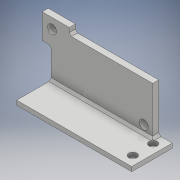
# Autodesk Inventor part: PingCover-y
Saved by Autodesk Inventor 2018 (Build 220112000, 112)
## iProperties
Created: 2018-08-25
Part Number: PingCover-y
Material: 一般
Document SubType Name: Modeling
Designer: shun2
Density: 1 g/cm^3
Appearance: 既定
Author: shun2
Autodesk Inventor part; units mm, degrees
ref_plane "YZ Plane" through (0, 0, 0) normal (1, 0, 0) x (0, 1, 0)
ref_plane "XZ Plane" through (0, 0, 0) normal (0, 1, 0) x (-1, 0, 0)
ref_plane "XY Plane" through (0, 0, 0) normal (0, 0, 1) x (1, 0, 0)
sketch "スケッチ1" plane through (0, 0, 0) normal (0, 0, 1) x (1, 0, 0)
  line L0 (0, 0) -> (51, 0)
  line L1 (51, 0) -> (51, 18)
  line L2 (51, 18) -> (0, 18)
  line L3 (0, 18) -> (0, 0)
  circle A0 centre (47, 13.5) radius 1.8
  circle A1 centre (47, 4.5) radius 1.8
  dimension "d0" = 51
  dimension "d1" = 18
  dimension "d4" = 3.6
  dimension "d5" = 13.5
  dimension "d6" = 4
  dimension "d7" = 3.6
  dimension "d8" = 4
  dimension "d9" = 4.5
  constraints: 8 end point, 2 centre point, 2 parallel, 1 horizontal, 1 perpendicular
  measures "d0" distance of L2.end L1.end
  measures "d1" distance of L1.end L0.end
  measures "d4" diameter of A0
  measures "d5" distance from line of L0 A0.centre
  measures "d6" distance from line of L1 A0.centre
  measures "d7" diameter of A1
  measures "d8" distance from line of L1 A1.centre
  measures "d9" distance from line of L0 A1.centre
extrude "押し出し2" add sketch "スケッチ1" along normal blind 2
sketch "スケッチ2" plane through (0, 0, 2) normal (0, 0, 1) x (1, 0, 0)
  line L0 (0, 18) -> (0, 0) projected
  line L1 (0, 18) -> (44, 18)
  line L2 (44, 18) -> (44, 15.3)
  line L3 (44, 15.3) -> (0, 15.3)
  line L4 (0, 15.3) -> (0, 18)
  dimension "d12" = 44
  dimension "d13" = 2.7
  constraints: 8 end point, 2 parallel, 1 horizontal, 1 perpendicular
  measures "d12" distance of L2.end L3.end
  measures "d13" distance of L1.end L2.end
extrude "押し出し3" add sketch "スケッチ2" along normal blind 21.3
sketch "スケッチ3" plane through (0, 15.3, 2) normal (0, -1, 0) x (1, 0, 0)
  circle A0 centre (41.1, 3.5) radius 2
  line L0 (44, 0) -> (44, 21.3) projected
  line L1 (44, 0) -> (0, 0) projected
  circle A1 centre (0.4, 19.8) radius 2
  point P0 (0, -2)
  dimension "d16" = 4
  dimension "d17" = 2.9
  dimension "d18" = 3.5
  dimension "d27" = 4
  dimension "d28" = 40.7
  dimension "d29" = 16.3
  constraints: 2 centre point
  measures "d16" diameter of A0
  measures "d17" distance from line of L0 A0.centre
  measures "d18" distance from line of L1 A0.centre
  measures "d27" diameter of A1
  measures "d28" horizontal distance of A0.centre A1.centre
  measures "d29" vertical distance of A0.centre A1.centre
sketch "スケッチ4" plane through (0, 15.3, 2) normal (0, -1, 0) x (1, 0, 0)
  line L0 (8, 13.3) -> (-4, 13.3)
  line L1 (-4, 13.3) -> (-4, 24.3)
  line L2 (-4, 24.3) -> (8, 24.3)
  line L3 (8, 24.3) -> (8, 13.3)
  line L4 (44, 0) -> (0, 0) projected
  line L5 (44, 0) -> (44, 21.3) projected
  line L6 (0, 21.3) -> (44, 21.3) projected
  line L7 (0, 0) -> (0, 21.3) projected
  point P0 (0, -2)
  dimension "d19" = 13.3
  dimension "d20" = 36
  dimension "d25" = 11
  dimension "d26" = 12
  constraints: 8 end point, 2 parallel, 1 horizontal, 1 perpendicular
  measures "d19" distance between parallel lines of L0 L4
  measures "d20" distance between parallel lines of L5 L3
  measures "d25" distance between parallel lines of L0 L2
  measures "d26" distance between parallel lines of L1 L3
extrude "押し出し4" add sketch "スケッチ4" against normal blind 2.7 contours L0 L7 L6 L3 | L0 L1 L2 L3 L6 L7
extrude "押し出し5" cut sketch "スケッチ3" against normal blind 2.75
sketch "スケッチ5" plane through (-4, 15.3, 26.3) normal (0, -1, 0) x (1, 0, 0)
  point P0 (4, -26.3)
sketch "スケッチ6" plane through (-4, 15.3, 26.3) normal (0, -1, 0) x (1, 0, 0)
  point P0 (4, -26.3)
sketch "スケッチ7" plane through (0, 15.3, 2) normal (0, -1, 0) x (1, 0, 0)
  point P0 (0, -2)
sketch "スケッチ8" plane through (0, 15.3, 2) normal (0, -1, 0) x (1, 0, 0)
  line L0 (44, 0) -> (44, 21.3) projected
  line L1 (44, 0) -> (45, 0)
  line L2 (45, 0) -> (45, 21.3)
  line L3 (45, 21.3) -> (44, 21.3)
  line L4 (44, 21.3) -> (44, 0)
  point P0 (0, -2)
  dimension "d35" = 1
  constraints: 8 end point, 2 parallel, 1 horizontal, 1 perpendicular
  measures "d35" distance of L3.end L2.end
extrude "押し出し6" add sketch "スケッチ8" against normal blind 2.7
chamfer "面取り2" distance 1 angle 45 2 edges at (0, 16.65, 15.3) (8, 16.65, 23.3)
chamfer "面取り3" distance 1 angle 45 2 edges at (22.5, 15.3, 2) (45, 16.65, 2)
